Autodesk Inventor part; units mm, degrees
(part 2 of 2)
  line L783 (1, 0.75) -> (1, 1.25)
  line L784 (1, 0) -> (7, 0) construction
  line L785 (7, 0) -> (1, 0) construction
  line L786 (-7, 11) -> (-1, 11)
  line L787 (-1, 11) -> (-1, -11)
  line L788 (-1, -11) -> (-7, -11)
  line L789 (-7, -11) -> (-7, 11)
  line L790 (-7, 1.25) -> (-4.8182, 1.25)
  line L791 (-4.8182, 1.25) -> (-4.8182, 0.75)
  line L792 (-4.8182, 0.75) -> (-7, 0.75)
  line L793 (-7, 0.75) -> (-7, 1.25)
  line L794 (-3.1818, 0.75) -> (-3.1818, 1.25)
  line L795 (-1, 0.75) -> (-3.1818, 0.75)
  line L796 (-3.1818, 1.25) -> (-1, 1.25)
  line L797 (-1, 1.25) -> (-1, 0.75)
  line L798 (-5.3636, -0.75) -> (-2.6364, -0.75)
  line L799 (-2.6364, -0.75) -> (-2.6364, -1.25)
  line L800 (-2.6364, -1.25) -> (-5.3636, -1.25)
  line L801 (-5.3636, -1.25) -> (-5.3636, -0.75)
  line L802 (-7, 0) -> (-1, 0) construction
  line L803 (-1, 0) -> (-7, 0) construction
  line L804 (-3.1818, -2.75) -> (-1, -2.75)
  line L805 (-1, -2.75) -> (-1, -3.25)
  line L806 (-1, -3.25) -> (-3.1818, -3.25)
  line L807 (-3.1818, -3.25) -> (-3.1818, -2.75)
  line L808 (-5.3636, -4.75) -> (-2.6364, -4.75)
  line L809 (-2.6364, -4.75) -> (-2.6364, -5.25)
  line L810 (-2.6364, -5.25) -> (-5.3636, -5.25)
  line L811 (-5.3636, -5.25) -> (-5.3636, -4.75)
  line L812 (-7, -2.75) -> (-4.8182, -2.75)
  line L813 (-4.8182, -2.75) -> (-4.8182, -3.25)
  line L814 (-4.8182, -3.25) -> (-7, -3.25)
  line L815 (-7, -3.25) -> (-7, -2.75)
  line L816 (-7, -4) -> (-1, -4) construction
  line L817 (-1, -4) -> (-7, -4) construction
  line L818 (-3.1818, -6.75) -> (-1, -6.75)
  line L819 (-1, -6.75) -> (-1, -7.25)
  line L820 (-1, -7.25) -> (-3.1818, -7.25)
  line L821 (-3.1818, -7.25) -> (-3.1818, -6.75)
  line L822 (-5.3636, -8.75) -> (-2.6364, -8.75)
  line L823 (-2.6364, -8.75) -> (-2.6364, -9.25)
  line L824 (-2.6364, -9.25) -> (-5.3636, -9.25)
  line L825 (-5.3636, -9.25) -> (-5.3636, -8.75)
  line L826 (-7, -6.75) -> (-4.8182, -6.75)
  line L827 (-4.8182, -6.75) -> (-4.8182, -7.25)
  line L828 (-4.8182, -7.25) -> (-7, -7.25)
  line L829 (-7, -7.25) -> (-7, -6.75)
  line L830 (-7, -8) -> (-1, -8) construction
  line L831 (-1, -8) -> (-7, -8) construction
  line L832 (-3.1818, 5.25) -> (-1, 5.25)
  line L833 (-1, 5.25) -> (-1, 4.75)
  line L834 (-1, 4.75) -> (-3.1818, 4.75)
  line L835 (-3.1818, 4.75) -> (-3.1818, 5.25)
  line L836 (-5.3636, 3.25) -> (-2.6364, 3.25)
  line L837 (-2.6364, 3.25) -> (-2.6364, 2.75)
  line L838 (-2.6364, 2.75) -> (-5.3636, 2.75)
  line L839 (-5.3636, 2.75) -> (-5.3636, 3.25)
  line L840 (-7, 5.25) -> (-4.8182, 5.25)
  line L841 (-4.8182, 5.25) -> (-4.8182, 4.75)
  line L842 (-4.8182, 4.75) -> (-7, 4.75)
  line L843 (-7, 4.75) -> (-7, 5.25)
  line L844 (-7, 4) -> (-1, 4) construction
  line L845 (-1, 4) -> (-7, 4) construction
  line L846 (-3.1818, 1.25) -> (-1, 1.25)
  line L847 (-1, 1.25) -> (-1, 0.75)
  line L848 (-1, 0.75) -> (-3.1818, 0.75)
  line L849 (-3.1818, 0.75) -> (-3.1818, 1.25)
  line L850 (-5.3636, -0.75) -> (-2.6364, -0.75)
  line L851 (-2.6364, -0.75) -> (-2.6364, -1.25)
  line L852 (-2.6364, -1.25) -> (-5.3636, -1.25)
  line L853 (-5.3636, -1.25) -> (-5.3636, -0.75)
  line L854 (-7, 1.25) -> (-4.8182, 1.25)
  line L855 (-4.8182, 1.25) -> (-4.8182, 0.75)
  line L856 (-4.8182, 0.75) -> (-7, 0.75)
  line L857 (-7, 0.75) -> (-7, 1.25)
  line L858 (-7, 0) -> (-1, 0) construction
  line L859 (-1, 0) -> (-7, 0) construction
  line L860 (-3.1818, -2.75) -> (-1, -2.75)
  line L861 (-1, -2.75) -> (-1, -3.25)
  line L862 (-1, -3.25) -> (-3.1818, -3.25)
  line L863 (-3.1818, -3.25) -> (-3.1818, -2.75)
  line L864 (-5.3636, -4.75) -> (-2.6364, -4.75)
  line L865 (-2.6364, -4.75) -> (-2.6364, -5.25)
  line L866 (-2.6364, -5.25) -> (-5.3636, -5.25)
  line L867 (-5.3636, -5.25) -> (-5.3636, -4.75)
  line L868 (-7, -2.75) -> (-4.8182, -2.75)
  line L869 (-4.8182, -2.75) -> (-4.8182, -3.25)
  line L870 (-4.8182, -3.25) -> (-7, -3.25)
  line L871 (-7, -3.25) -> (-7, -2.75)
  line L872 (-7, -4) -> (-1, -4) construction
  line L873 (-1, -4) -> (-7, -4) construction
  line L874 (-3.1818, 9.25) -> (-1, 9.25)
  line L875 (-1, 9.25) -> (-1, 8.75)
  line L876 (-1, 8.75) -> (-3.1818, 8.75)
  line L877 (-3.1818, 8.75) -> (-3.1818, 9.25)
  line L878 (-5.3636, 7.25) -> (-2.6364, 7.25)
  line L879 (-2.6364, 7.25) -> (-2.6364, 6.75)
  line L880 (-2.6364, 6.75) -> (-5.3636, 6.75)
  line L881 (-5.3636, 6.75) -> (-5.3636, 7.25)
  line L882 (-7, 9.25) -> (-4.8182, 9.25)
  line L883 (-4.8182, 9.25) -> (-4.8182, 8.75)
  line L884 (-4.8182, 8.75) -> (-7, 8.75)
  line L885 (-7, 8.75) -> (-7, 9.25)
  line L886 (-7, 8) -> (-1, 8) construction
  line L887 (-1, 8) -> (-7, 8) construction
  line L888 (-3.1818, 5.25) -> (-1, 5.25)
  line L889 (-1, 5.25) -> (-1, 4.75)
  line L890 (-1, 4.75) -> (-3.1818, 4.75)
  line L891 (-3.1818, 4.75) -> (-3.1818, 5.25)
  line L892 (-5.3636, 3.25) -> (-2.6364, 3.25)
  line L893 (-2.6364, 3.25) -> (-2.6364, 2.75)
  line L894 (-2.6364, 2.75) -> (-5.3636, 2.75)
  line L895 (-5.3636, 2.75) -> (-5.3636, 3.25)
  line L896 (-7, 5.25) -> (-4.8182, 5.25)
  line L897 (-4.8182, 5.25) -> (-4.8182, 4.75)
  line L898 (-4.8182, 4.75) -> (-7, 4.75)
  line L899 (-7, 4.75) -> (-7, 5.25)
  line L900 (-7, 4) -> (-1, 4) construction
  line L901 (-1, 4) -> (-7, 4) construction
  line L902 (-3.1818, 1.25) -> (-1, 1.25)
  line L903 (-1, 1.25) -> (-1, 0.75)
  line L904 (-1, 0.75) -> (-3.1818, 0.75)
  line L905 (-3.1818, 0.75) -> (-3.1818, 1.25)
  line L906 (-5.3636, -0.75) -> (-2.6364, -0.75)
  line L907 (-2.6364, -0.75) -> (-2.6364, -1.25)
  line L908 (-2.6364, -1.25) -> (-5.3636, -1.25)
  line L909 (-5.3636, -1.25) -> (-5.3636, -0.75)
  line L910 (-7, 1.25) -> (-4.8182, 1.25)
  line L911 (-4.8182, 1.25) -> (-4.8182, 0.75)
  line L912 (-4.8182, 0.75) -> (-7, 0.75)
  line L913 (-7, 0.75) -> (-7, 1.25)
  line L914 (-7, 0) -> (-1, 0) construction
  line L915 (-1, 0) -> (-7, 0) construction
  line L916 (-3.1818, -10.75) -> (-1, -10.75)
  line L917 (-1, -10.75) -> (-1, -11.25)
  line L918 (-1, -11.25) -> (-3.1818, -11.25)
  line L919 (-3.1818, -11.25) -> (-3.1818, -10.75)
  line L920 (-5.3636, -12.75) -> (-2.6364, -12.75)
  line L921 (-2.6364, -12.75) -> (-2.6364, -13.25)
  line L922 (-2.6364, -13.25) -> (-5.3636, -13.25)
  line L923 (-5.3636, -13.25) -> (-5.3636, -12.75)
  line L924 (-7, -10.75) -> (-4.8182, -10.75)
  line L925 (-4.8182, -10.75) -> (-4.8182, -11.25)
  line L926 (-4.8182, -11.25) -> (-7, -11.25)
  line L927 (-7, -11.25) -> (-7, -10.75)
  line L928 (-7, -12) -> (-1, -12) construction
  line L929 (-1, -12) -> (-7, -12) construction
  line L930 (-3.1818, -6.75) -> (-1, -6.75)
  line L931 (-1, -6.75) -> (-1, -7.25)
  line L932 (-1, -7.25) -> (-3.1818, -7.25)
  line L933 (-3.1818, -7.25) -> (-3.1818, -6.75)
  line L934 (-5.3636, -8.75) -> (-2.6364, -8.75)
  line L935 (-2.6364, -8.75) -> (-2.6364, -9.25)
  line L936 (-2.6364, -9.25) -> (-5.3636, -9.25)
  line L937 (-5.3636, -9.25) -> (-5.3636, -8.75)
  line L938 (-7, -6.75) -> (-4.8182, -6.75)
  line L939 (-4.8182, -6.75) -> (-4.8182, -7.25)
  line L940 (-4.8182, -7.25) -> (-7, -7.25)
  line L941 (-7, -7.25) -> (-7, -6.75)
  line L942 (-7, -8) -> (-1, -8) construction
  line L943 (-1, -8) -> (-7, -8) construction
  line L944 (-3.1818, -2.75) -> (-1, -2.75)
  line L945 (-1, -2.75) -> (-1, -3.25)
  line L946 (-1, -3.25) -> (-3.1818, -3.25)
  line L947 (-3.1818, -3.25) -> (-3.1818, -2.75)
  line L948 (-5.3636, -4.75) -> (-2.6364, -4.75)
  line L949 (-2.6364, -4.75) -> (-2.6364, -5.25)
  line L950 (-2.6364, -5.25) -> (-5.3636, -5.25)
  line L951 (-5.3636, -5.25) -> (-5.3636, -4.75)
  line L952 (-7, -2.75) -> (-4.8182, -2.75)
  line L953 (-4.8182, -2.75) -> (-4.8182, -3.25)
  line L954 (-4.8182, -3.25) -> (-7, -3.25)
  line L955 (-7, -3.25) -> (-7, -2.75)
  line L956 (-7, -4) -> (-1, -4) construction
  line L957 (-1, -4) -> (-7, -4) construction
  line L958 (-3.1818, 13.25) -> (-1, 13.25)
  line L959 (-1, 13.25) -> (-1, 12.75)
  line L960 (-1, 12.75) -> (-3.1818, 12.75)
  line L961 (-3.1818, 12.75) -> (-3.1818, 13.25)
  line L962 (-5.3636, 11.25) -> (-2.6364, 11.25)
  line L963 (-2.6364, 11.25) -> (-2.6364, 10.75)
  line L964 (-2.6364, 10.75) -> (-5.3636, 10.75)
  line L965 (-5.3636, 10.75) -> (-5.3636, 11.25)
  line L966 (-7, 13.25) -> (-4.8182, 13.25)
  line L967 (-4.8182, 13.25) -> (-4.8182, 12.75)
  line L968 (-4.8182, 12.75) -> (-7, 12.75)
  line L969 (-7, 12.75) -> (-7, 13.25)
  line L970 (-7, 12) -> (-1, 12) construction
  line L971 (-1, 12) -> (-7, 12) construction
  line L972 (-3.1818, 9.25) -> (-1, 9.25)
  line L973 (-1, 9.25) -> (-1, 8.75)
  line L974 (-1, 8.75) -> (-3.1818, 8.75)
  line L975 (-3.1818, 8.75) -> (-3.1818, 9.25)
  line L976 (-5.3636, 7.25) -> (-2.6364, 7.25)
  line L977 (-2.6364, 7.25) -> (-2.6364, 6.75)
  line L978 (-2.6364, 6.75) -> (-5.3636, 6.75)
  line L979 (-5.3636, 6.75) -> (-5.3636, 7.25)
  line L980 (-7, 9.25) -> (-4.8182, 9.25)
  line L981 (-4.8182, 9.25) -> (-4.8182, 8.75)
  line L982 (-4.8182, 8.75) -> (-7, 8.75)
  line L983 (-7, 8.75) -> (-7, 9.25)
  line L984 (-7, 8) -> (-1, 8) construction
  line L985 (-1, 8) -> (-7, 8) construction
  line L986 (-3.1818, 5.25) -> (-1, 5.25)
  line L987 (-1, 5.25) -> (-1, 4.75)
  line L988 (-1, 4.75) -> (-3.1818, 4.75)
  line L989 (-3.1818, 4.75) -> (-3.1818, 5.25)
  line L990 (-5.3636, 3.25) -> (-2.6364, 3.25)
  line L991 (-2.6364, 3.25) -> (-2.6364, 2.75)
  line L992 (-2.6364, 2.75) -> (-5.3636, 2.75)
  line L993 (-5.3636, 2.75) -> (-5.3636, 3.25)
  line L994 (-7, 5.25) -> (-4.8182, 5.25)
  line L995 (-4.8182, 5.25) -> (-4.8182, 4.75)
  line L996 (-4.8182, 4.75) -> (-7, 4.75)
  line L997 (-7, 4.75) -> (-7, 5.25)
  line L998 (-7, 4) -> (-1, 4) construction
  line L999 (-1, 4) -> (-7, 4) construction
  line L1000 (-3.1818, 1.25) -> (-1, 1.25)
  line L1001 (-1, 1.25) -> (-1, 0.75)
  line L1002 (-1, 0.75) -> (-3.1818, 0.75)
  line L1003 (-3.1818, 0.75) -> (-3.1818, 1.25)
  line L1004 (-5.3636, -0.75) -> (-2.6364, -0.75)
  line L1005 (-2.6364, -0.75) -> (-2.6364, -1.25)
  line L1006 (-2.6364, -1.25) -> (-5.3636, -1.25)
  line L1007 (-5.3636, -1.25) -> (-5.3636, -0.75)
  line L1008 (-7, 1.25) -> (-4.8182, 1.25)
  line L1009 (-4.8182, 1.25) -> (-4.8182, 0.75)
  line L1010 (-4.8182, 0.75) -> (-7, 0.75)
  line L1011 (-7, 0.75) -> (-7, 1.25)
  line L1012 (-7, 0) -> (-1, 0) construction
  line L1013 (-1, 0) -> (-7, 0) construction
  line L1014 (-7.725, 16) -> (-4.675, 16)
  line L1015 (-4.675, 16) -> (-4.675, 12.925)
  line L1016 (-4.675, 12.925) -> (-7.725, 12.925)
  line L1017 (-7.725, 12.925) -> (-7.725, 16)
  line L1018 (0, 18.7013) -> (0, 11.7377) construction
  line L1019 (-1.525, 16) -> (1.525, 16)
  line L1020 (1.525, 16) -> (1.525, 12.925)
  line L1021 (1.525, 12.925) -> (-1.525, 12.925)
  line L1022 (-1.525, 12.925) -> (-1.525, 16)
  line L1023 (4.675, 16) -> (7.725, 16)
  line L1024 (7.725, 16) -> (7.725, 12.925)
  line L1025 (7.725, 12.925) -> (4.675, 12.925)
  line L1026 (4.675, 12.925) -> (4.675, 16)
  line L1027 (0, 12.925) -> (0, 12.0116) construction
  point P0 (0, 0)
  point P1 (0, 25)
  point P2 (25, 0)
  point P3 (0, 16)
  point P4 (-4, -11)
  point P5 (-4, -11)
  point P6 (4, -11)
  point P7 (4, -11)
  dimension "d76" = 6
  dimension "d89" = 3
  dimension "d90" = 3
  dimension "d91" = 2
  dimension "d0" = 50
  dimension "d1" = 50
  dimension "d16" = 6
  dimension "d19" = 6
  dimension "d21" = 5
  dimension "d75" = 3
  dimension "d94" = 3
  dimension "d95" = 2
  dimension "d96" = 6
  dimension "d97" = 6
  dimension "d101" = 32
  dimension "d114" = 1
  dimension "d115" = 1
  dimension "d116" = 1
  constraints: 84 end point, 23 horizontal, 20 parallel, 11 perpendicular, 10 vertical, 5 equal length, 5 midpoint, 3 centre point, 3 collinear, 2 coincident, 2 point on line, 2 vertical alignment, 1 horizontal alignment, 4 other
  measures "d0" distance of L1.end L2.end
  measures "d1" distance of L0.end L1.end
  measures "d16" distance between parallel lines of L12 L10
  measures "d19" distance between parallel lines of L4 L6
  measures "d21" distance between parallel lines of L32 L30
  measures "d75" distance between parallel lines of L33 L15
  measures "d94" distance between parallel lines of L30 L12
  measures "d95" distance between parallel lines of L6 L16
  measures "d96" distance of L35.end L36.end
  measures "d97" distance of L39.end L40.end
  measures "d101" distance of L30.start L30.end
  measures "d114" diameter of A0
  measures "d115" diameter of A1
  measures "d116" diameter of A2
extrude "Extrusion2" add sketch "Sketch1" along normal blind 3.1 contours L7 L6 L5 L4 L70 L69 L72 L66 L65 L68 L61 L60 L63 | L37 L926 L925 L34 L919 L918 L35 L6 | L37 L34 L925 L926 | L41 L698 L697 L38 L691 L690 L39 L6 | L918 L919 L34 L35 | L789 L924 L925 L34 | L41 L38 L697 L698 | L34 L919 L916 L787 | L925 L924 L789 L828 L827 L826 L814 L813 L812 L792 L791 L790 L842 L841 L840 L884 L883 L882 L32 L965 L964 L963 L787 L874 L877 L876 L832 L835 L834 L796 L794 L795 L804 L807 L806 L818 L821 L820 L916 L919 L34 | L690 L691 L38 L39 | L561 L696 L697 L38 | L38 L691 L688 L559 | L697 L696 L561 L600 L599 L598 L586 L585 L584 L564 L563 L562 L614 L613 L612 L656 L655 L654 L32 L737 L736 L735 L559 L646 L649 L648 L604 L607 L606 L568 L566 L567 L576 L579 L578 L590 L593 L592 L688 L691 L38 | L32 L279 L278 L281 L33 L284 L283 L282 L30 L1017 L1016 L969 L968 L967 L1015 L1022 L958 L961 L960 L959 L1021 L741 L740 L739 L738 L1020 L1026 L1025 L733 L732 L731 L1024 L31 L502 L505 L504 L507 L506 L509 L735 L734 L737 L963 L962 L965 | L103 L190 L193 L192 L148 L151 L150 L112 L110 L111 L120 L123 L122 L134 L137 L136 L232 L235 L20 L241 L240 L105 L144 L143 L142 L130 L129 L128 L108 L107 L106 L158 L157 L156 L200 L199 L198 L32 L281 L280 L279 | L965 L962 L963 L32 | L32 L963 L964 L965 | L279 L280 L281 L32 | L32 L281 L278 L279 | L737 L734 L735 L32 | L32 L735 L736 L737 | L32 L509 L508 L507 L331 L418 L421 L420 L376 L379 L378 L340 L338 L339 L348 L351 L350 L362 L365 L364 L460 L463 L28 L469 L468 L333 L372 L371 L370 L358 L357 L356 L336 L335 L334 L386 L385 L384 L428 L427 L426 | L509 L506 L507 L32 | L32 L507 L508 L509 | L33 L282 L283 L284 | L504 L505 L502 L31 | L1016 L967 L968 L969 | L1022 L1021 L959 L960 L961 L958 | L738 L739 L740 L741 L1021 L1020 | L103 L20 L235 L232 | L731 L732 L733 L1025 | L19 L234 L235 L20 | L19 L18 L15 L20 L243 L242 L241 L235 L234 | L468 L469 L28 L333 | L240 L241 L20 L105 | L241 L242 L243 L20 | L28 L469 L470 L27 | L16 L17 L77 L76 L75 L82 L81 L80 L86 L85 L84 L12 L15 | L470 L469 L28 L463 L462 L461 L23 L26 L27 | L331 L28 L463 L460 | L28 L461 L462 L463 | L12 L13 L10 L49 L48 L47 L54 L53 L52 L58 L57 L56 L11 | L23 L12 L25 L98 L97 L100 L94 L93 L96 L89 L88 L91 L24 | L236 L237 L238 L239 | L274 L275 L276 L277 | L464 L465 L466 L467 | L510 L511 L512 L513 | L692 L693 L694 L695 | L920 L921 L922 L923
equation "\"d2\" = mat - kerf"
equation "\"d3\" = mat - 0.5 * kerf"
equation "\"d22\" = flex_w"
equation "\"d24\" = 0.363636 * flex_w"
equation "\"d27\" = 0.636364 * flex_w"
equation "\"d32\" = 0.272727 * flex_w"
equation "\"d33\" = 0.454545 * flex_w"
equation "\"d41\" = line_w"
equation "\"d42\" = line_w"
equation "\"d43\" = line_sp"
equation "\"d93\" = flex_h"
equation "\"d89\" = flex_sp"
equation "\"d90\" = flex_sp"
equation "\"d16\" = structure_w"
equation "\"d19\" = structure_w"
equation "\"structure_w\" = 6"
equation "\"structure_sp\" = 8"
equation "\"flex_w\" = 6"
equation "\"line_w\" = 0.5"
equation "\"line_sp\" = 1.5"
equation "\"flex_sp\" = 3"
equation "\"mat\" = 3.1"
equation "\"kerf\" = 0.05"
equation "\"flex_h\" = 22"
body "Solid2"
